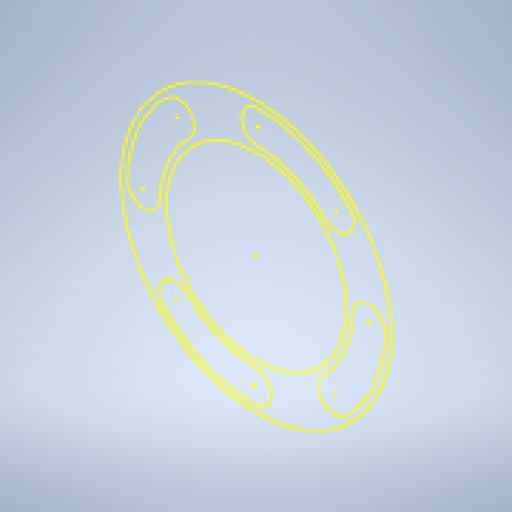
# Autodesk Inventor part: Clutch_Pin
Saved by Autodesk Inventor 2024.3 (Build 283343000, 343)
## iProperties
Created: 2024-11-08
Part Number: Clutch_Pin
Material: Generic
Document SubType Name: Modeling
Designer: wszaf
Density: 1 g/cm^3
Appearance: Default
Author: wszaf
Autodesk Inventor part; units mm, degrees
ref_plane "YZ Plane" through (0, 0, 0) normal (1, 0, 0) x (0, 1, 0)
ref_plane "XZ Plane" through (0, 0, 0) normal (0, 1, 0) x (-1, 0, 0)
ref_plane "XY Plane" through (0, 0, 0) normal (0, 0, 1) x (1, 0, 0)
sketch "Sketch1" plane through (0, 0, 0) normal (0, 0, 1) x (1, 0, 0)
  arc A0 (-6.1759, -5.9849) -> (-0.135, -8.5989) centre (0, 0) ccw projected
  arc A1 (-0.135, -8.5989) -> (-0.1005, -6.3992) centre (-0.1178, -7.4991) ccw projected
  arc A2 (-4.596, -4.4539) -> (-0.1005, -6.3992) centre (0, 0) ccw projected
  arc A3 (-4.596, -4.4539) -> (-6.1759, -5.9849) centre (-5.3859, -5.2194) ccw projected
  arc A4 (5.9849, -6.1759) -> (8.5989, -0.135) centre (0, 0) ccw projected
  arc A5 (8.5989, -0.135) -> (6.3992, -0.1005) centre (7.4991, -0.1178) ccw projected
  arc A6 (4.4539, -4.596) -> (6.3992, -0.1005) centre (0, 0) ccw projected
  arc A7 (4.4539, -4.596) -> (5.9849, -6.1759) centre (5.2194, -5.3859) ccw projected
  arc A8 (6.1759, 5.9849) -> (0.135, 8.5989) centre (0, 0) ccw projected
  arc A9 (0.135, 8.5989) -> (0.1005, 6.3992) centre (0.1178, 7.4991) ccw projected
  arc A10 (4.596, 4.4539) -> (0.1005, 6.3992) centre (0, 0) ccw projected
  arc A11 (4.596, 4.4539) -> (6.1759, 5.9849) centre (5.3859, 5.2194) ccw projected
  arc A12 (-5.9849, 6.1759) -> (-8.5989, 0.135) centre (0, 0) ccw projected
  arc A13 (-8.5989, 0.135) -> (-6.3992, 0.1005) centre (-7.4991, 0.1178) ccw projected
  arc A14 (-4.4539, 4.596) -> (-6.3992, 0.1005) centre (0, 0) ccw projected
  arc A15 (-4.4539, 4.596) -> (-5.9849, 6.1759) centre (-5.2194, 5.3859) ccw projected
  circle A16 centre (0, 0) radius 9 projected
  circle A17 centre (0, 0) radius 6 projected
  point P0 (0, 0)
extrude "Extrusion1" add sketch "Sketch1" along normal blind 11.6 contours A11 A10 A9 A8
equation "\"Fit_Loose\" = 0.4"
body "Solid1"
